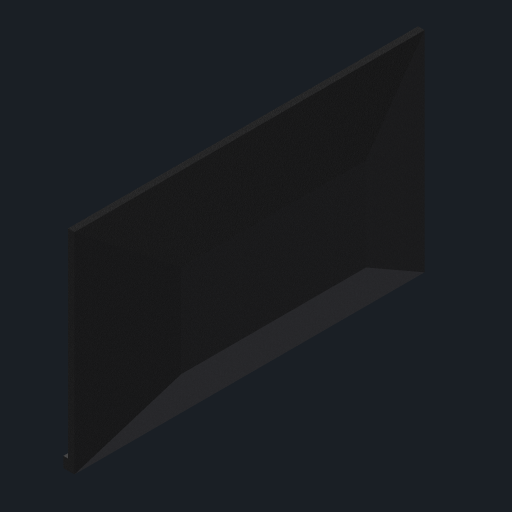
# Autodesk Inventor part: PANTALLA
Saved by Autodesk Inventor 2024.3 (Build 283343000, 343)
## iProperties
Created: 2024-07-02
Part Number: PANTALLA
Material: Steel, Mild, Welded
Document SubType Name: Modeling
Designer: Niler
Density: 7.85 g/cm^3
Appearance: Weld - Steel Mild
Author: Niler
Autodesk Inventor part; units mm, degrees
ref_plane "YZ Plane" through (0, 0, 0) normal (1, 0, 0) x (0, 1, 0)
ref_plane "XZ Plane" through (0, 0, 0) normal (0, 1, 0) x (-1, 0, 0)
sketch "Sketch1" plane through (0, 0, 0) normal (1, 0, 0) x (0, 1, 0)
  line L0 (-161.65, 269.7) -> (161.65, 269.7)
  line L1 (161.65, 269.7) -> (161.65, -269.7)
  line L2 (161.65, -269.7) -> (-161.65, -269.7)
  line L3 (-161.65, -269.7) -> (-161.65, 269.7)
  line L4 (-161.65, 269.7) -> (161.65, -269.7) construction
  line L5 (161.65, 269.7) -> (-161.65, -269.7) construction
  point P0 (0, 0)
  dimension "d0" = 323.3
  dimension "d1" = 539.4
  constraints: 12 end point, 2 midpoint, 2 parallel, 1 horizontal, 1 perpendicular
  measures "d0" distance of L1.end L2.end
  measures "d1" distance of L0.end L1.end
extrude "Extrusion1" add sketch "Sketch1" along normal blind 10
ref_plane "Work Plane1" through (47, 0, 0) normal (1, 0, 0) x (0, 0, -1)
sketch "Sketch2" plane through (47, 0, 0) normal (1, 0, 0) x (0, 0, -1)
  line L0 (-142.5, 69.9526) -> (142.5, 69.9526)
  line L1 (142.5, 69.9526) -> (142.5, -73.0474)
  line L2 (142.5, -73.0474) -> (-142.5, -73.0474)
  line L3 (-142.5, -73.0474) -> (-142.5, 69.9526)
  line L4 (-142.5, 69.9526) -> (142.5, -73.0474) construction
  line L5 (142.5, 69.9526) -> (-142.5, -73.0474) construction
  point P0 (0, 0)
  point P1 (0, -1.5474)
  dimension "d5" = 285
  dimension "d6" = 143
  constraints: 12 end point, 2 midpoint, 2 parallel, 1 horizontal, 1 perpendicular, 1 vertical alignment
  measures "d5" distance of L1.end L2.end
  measures "d6" distance of L0.end L1.end
sketch "Sketch3" plane through (10, 0, 0) normal (1, 0, 0) x (0, 0, -1)
  line L0 (269.7, -161.65) -> (269.7, 161.65) projected
  line L1 (269.7, 161.65) -> (-269.7, 161.65) projected
  line L2 (-269.7, 161.65) -> (-269.7, -161.65) projected
  line L3 (-269.7, -161.65) -> (269.7, -161.65) projected
  point P0 (0, 0)
loft "Loft1" add profiles "Sketch2" section 1 edges at (10, 0, -269.7) (10, 161.65, 0) (10, 0, 269.7) (10, -161.65, 0)
sketch "Sketch4" plane through (0, 0, 0) normal (-1, 0, 0) x (0, 0, 1)
  line L0 (-269.7, -161.65) -> (-269.7, 161.65) projected
  line L1 (269.7, -161.65) -> (-269.7, -161.65) projected
  line L2 (269.7, 161.65) -> (269.7, -161.65) projected
  line L3 (-269.7, 161.65) -> (269.7, 161.65) projected
  line L4 (-269.7, -161.65) -> (-269.7, 161.65) projected
  line L5 (-269.7, -145.2634) -> (269.7, -145.2634)
  point P0 (0, 0)
  constraints: 2 end point, 2 point on line, 1 perpendicular
extrude "Extrusion2" add sketch "Sketch4" along normal blind 7 contours L0 L5 L2 L1
body "Solid1"
